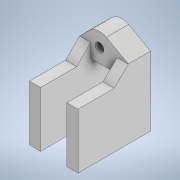
# Autodesk Inventor part: Part1
Saved by Autodesk Inventor 2022 (Build 260153000, 153)
## iProperties
Created: 2021-04-05
Part Number: Part1
Material: Generic
Document SubType Name: Modeling
Designer: chris
Density: 1 g/cm^3
Appearance: Default
Author: chris
Autodesk Inventor part; units mm, degrees
ref_plane "YZ Plane" through (0, 0, 0) normal (1, 0, 0) x (0, 1, 0)
ref_plane "XZ Plane" through (0, 0, 0) normal (0, 1, 0) x (-1, 0, 0)
ref_plane "XY Plane" through (0, 0, 0) normal (0, 0, 1) x (1, 0, 0)
sketch "Sketch1" plane through (0, 0, 0) normal (0, 0, 1) x (1, 0, 0)
  circle A0 centre (0, 0) radius 3.175
  circle A1 centre (0, 0) radius 1.0033
  line L0 (0.1283, -1.7725) -> (1.8783, -1.7725)
  line L1 (1.0033, 0) -> (1.0033, -0.8261)
  line L2 (-1.9967, -1.7725) -> (4.0033, -1.7725)
  line L3 (-1.9967, -1.7725) -> (-1.9967, -15.7725)
  line L4 (-1.9967, -15.7725) -> (-4.5367, -15.7725)
  line L5 (-4.5367, -15.7725) -> (-4.5367, 0)
  line L6 (-4.5367, 0) -> (-2.222, 2.2679)
  line L7 (4.0033, -1.7725) -> (4.0033, -15.7725)
  line L8 (4.0033, -15.7725) -> (6.5433, -15.7725)
  line L9 (6.5433, -15.7725) -> (6.5433, 0)
  line L10 (6.5433, 0) -> (1.5406, 2.7762)
  line L11 (0, -3.175) -> (4.0033, -3.175)
  line L12 (0, -3.175) -> (-1.9967, -3.175)
  point P0 (1.0033, -1.7725)
  point P1 (-2.4117, -2.065)
  point P2 (3.1483, -0.4109)
  point P3 (-1.1417, -15.7725)
  point P4 (2.2816, 2.208)
  point P5 (1.0033, -1.7725)
  point P6 (1.5406, 2.7762)
  dimension "d1" = 2.0066
  dimension "d0" = 6.35
  dimension "d2" = 1.75
  dimension "d10" = 6
  dimension "d11" = 2.54
  dimension "d12" = 2.54
  constraints: 26 end point, 5 point on circle, 4 perpendicular, 4 point on line, 3 coincident, 3 horizontal, 3 tangent, 3 vertical, 2 midpoint, 1 centre point, 1 horizontal alignment, 1 vertical alignment, 2 other
  measures "d0" diameter of A0
  measures "d2" distance of L0.start L0.end
  measures "d10" distance of L2.start L2.end
  measures "d11" distance of L3.end L4.end
  measures "d12" distance of L7.end L8.end
extrude "Extrusion2" add sketch "Sketch1" along normal blind 16.51
sketch "Sketch2" plane through (0, 0, 16.51) normal (0, 0, 1) x (1, 0, 0)
  arc A0 (1.5406, 2.7762) -> (-2.222, 2.2679) centre (0, 0) ccw projected
  line L0 (-2.222, 2.2679) -> (-4.5367, 0) projected
  line L1 (-4.5367, 0) -> (-4.5367, -15.7725) projected
  line L2 (-4.5367, -15.7725) -> (-1.9967, -15.7725) projected
  line L3 (-1.9967, -15.7725) -> (-1.9967, -3.175) projected
  line L4 (-1.9967, -3.175) -> (4.0033, -3.175) projected
  line L5 (4.0033, -3.175) -> (4.0033, -15.7725) projected
  line L6 (4.0033, -15.7725) -> (6.5433, -15.7725) projected
  line L7 (6.5433, -15.7725) -> (6.5433, 0) projected
  line L8 (6.5433, 0) -> (1.5406, 2.7762) projected
  circle A1 centre (0, 0) radius 1.0033 projected
  line L9 (-4.5367, 0) -> (-4.5367, -15.7725) projected
  line L10 (-4.5367, -3.175) -> (6.5433, -3.175)
  line L11 (6.5433, -15.7725) -> (6.5433, 0) projected
  point P0 (-1.9967, -3.175)
  constraints: 2 end point, 2 point on line, 1 horizontal
extrude "Extrusion3" cut sketch "Sketch2" against normal blind 11.43 contours L8 L7 L10 L4 L1 L0 A0
chamfer "Chamfer1" distance 3.175 angle 45 2 edges at (5.2733, -3.175, 5.08) (-3.2667, -3.175, 5.08)
body "Solid2"
